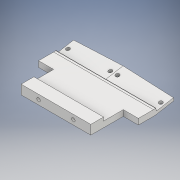
# Autodesk Inventor part: 앞뒷면PSD받침대_수정
Saved by Autodesk Inventor 2017 (Build 210142000, 142)
## iProperties
Part Number: 앞뒷면PSD받침대_수정
Material: ABS 플라스틱
Document SubType Name: Modeling
Designer: minom
Mass: 12.9687 g
Surface Area: 93.8696 cm^2
Volume: 12.2346 cm^3
Density: 1.06 g/cm^3
Appearance: 매끄러움 - 흰색
Author: minom
Autodesk Inventor part; units mm, degrees
ref_plane "YZ Plane" through (0, 0, 0) normal (1, 0, 0) x (0, 1, 0)
ref_plane "XZ Plane" through (0, 0, 0) normal (0, 1, 0) x (-1, 0, 0)
ref_plane "XY Plane" through (0, 0, 0) normal (0, 0, 1) x (1, 0, 0)
sketch "스케치1" plane through (0, 0, 0) normal (0, 0, 1) x (1, 0, 0)
  line L0 (0, 0) -> (60, 0)
  line L1 (60, 0) -> (60, 25)
  line L2 (60, 55) -> (0, 55)
  line L3 (0, 25) -> (0, 0)
  line L4 (-13, 55) -> (73, 55)
  line L5 (73, 55) -> (73, 25)
  line L6 (-13, 25) -> (-13, 55)
  line L7 (73, 25) -> (60, 25)
  line L8 (0, 25) -> (-13, 25)
  dimension "d0" = 60
  dimension "d1" = 55
  dimension "d3" = 86
  dimension "d4" = 30
  dimension "d5" = 13
  constraints: 18 end point, 5 parallel, 2 horizontal, 2 perpendicular
  measures "d0" distance of L2.end L2.start
  measures "d1" distance of L2.start L0.end
  measures "d3" distance of L5.end L6.start
  measures "d4" distance of L4.end L5.end
  measures "d5" distance between parallel lines of L3 L6
extrude "돌출1" add sketch "스케치1" along normal blind 8
sketch "스케치2" plane through (0, 0, 8) normal (0, 0, 1) x (1, 0, 0)
  line L0 (0, 0) -> (60, 0) projected
  line L1 (60, 0) -> (60, 25) projected
  line L2 (60, 25) -> (73, 25) projected
  line L3 (73, 25) -> (73, 55) projected
  line L4 (73, 55) -> (-13, 55) projected
  line L5 (-13, 55) -> (-13, 25) projected
  line L6 (-13, 25) -> (0, 25) projected
  line L7 (0, 25) -> (0, 0) projected
  line L8 (0, 25) -> (0, 0) projected
  line L9 (0, 8) -> (60, 8)
  line L10 (60, 8) -> (60, 0)
  line L11 (60, 0) -> (0, 0)
  line L12 (0, 0) -> (0, 8)
  dimension "d9" = 8
  dimension "d10" = 0
  constraints: 8 end point, 2 parallel, 2 point on line, 1 horizontal, 1 perpendicular
  measures "d9" distance of L9.end L10.end
  measures "d10" distance between parallel lines of L0 L11
extrude "돌출2" cut sketch "스케치2" against normal blind 3 contours L7 L6 L5 L4 L3 L2 L1 L9
sketch "스케치4" plane through (0, 0, 0) normal (0, -1, 0) x (1, 0, 0)
  line L0 (0, 0) -> (60, 0) projected
  line L1 (60, 0) -> (60, 8) projected
  line L2 (0, 8) -> (60, 8) projected
  line L3 (0, 0) -> (0, 8) projected
  circle A0 centre (45, 4) radius 1.5
  circle A1 centre (15, 4) radius 1.5
  dimension "d15" = 3
  dimension "d16" = 3
  dimension "d17" = 4
  dimension "d18" = 15
  dimension "d19" = 4
  dimension "d20" = 15
  constraints: 2 centre point
  measures "d15" diameter of A0
  measures "d16" diameter of A1
  measures "d17" distance from line of L0 A0.centre
  measures "d18" distance from line of L1 A0.centre
  measures "d19" distance from line of L2 A1.centre
  measures "d20" distance from line of L3 A1.centre
extrude "돌출4" cut sketch "스케치4" against normal blind 6 contours A0 | A1
sketch "스케치10" plane through (0, 0, 5) normal (0, 0, 1) x (1, 0, 0)
  line L0 (-10, 38) -> (70, 38)
  line L1 (60, 8) -> (0, 8) projected
  point P0 (0, 0)
  dimension "d42" = 30
  constraints: 2 end point, 1 horizontal
  measures "d42" distance between parallel lines of L1 L0
bend part "굽힘1" radius 10 angle 10 line through (-10, 38, 5) along (1, 0, 0) centre toward (0, 0, 1) moving side (0, 1, 0) both sides no
sketch "스케치11" plane through (-13, 54.7594, 7.8009) normal (0, 0.9848078, 0.1736482) x (1, 0, 0)
  line L0 (0, 0) -> (86, 0) projected
  line L1 (86, 5) -> (86, 0) projected
  line L2 (86, 5) -> (0, 5) projected
  line L3 (0, 5) -> (0, 0) projected
  line L4 (0, 2.5) -> (43, 0)
  line L5 (0, 0) -> (86, 0) projected
  line L6 (73, 2.5147) -> (86, 2.5147) projected
  line L7 (86, 2.5147) -> (43, 0)
  line L8 (43, 0) -> (43, 2.5)
  line L9 (86, 5) -> (0, 5) projected
  line L10 (86, 5) -> (43, 2.5)
  line L11 (0, 5) -> (43, 2.5)
  point P0 (13, -1.8265)
  constraints: 10 end point, 2 midpoint, 1 parallel, 1 perpendicular
extrude "돌출7" cut sketch "스케치11" against normal blind 15 contours L3 L4 L0 | L7 L1 L0 | L11 L2 L10
sketch "스케치12" plane through (30, 54.7594, 7.8009) normal (0.0583814, -0.173352, 0.983128) x (0.9982944, 0.0101378, -0.0574945)
  line L0 (0, 0) -> (43.0735, 0) projected
  line L1 (0, -15) -> (0, 0) projected
  line L2 (0, -15) -> (43.0735, -15) projected
  line L3 (43.0735, 0) -> (43.0735, -15) projected
  circle A0 centre (3.0735, -8) radius 1.6
  circle A1 centre (40.0735, -8) radius 1.6
  point P0 (-30.0555, -55.2821)
  dimension "d47" = 3.2
  dimension "d48" = 3.2
  dimension "d49" = 8
  dimension "d50" = 7
  dimension "d51" = 37
  dimension "d52" = 3
  constraints: 2 centre point
  measures "d47" diameter of A0
  measures "d48" diameter of A1
  measures "d49" distance from line of L0 A0.centre
  measures "d50" distance from line of L2 A1.centre
  measures "d51" distance of A1.centre A0.centre
  measures "d52" distance from line of L3 A1.centre
sketch "스케치13" plane through (-13, 55.1935, 5.3388) normal (-0.0580415, -0.1733554, 0.9831475) x (0.9983142, -0.0100788, 0.0571597)
  circle A0 centre (3, -8) radius 1.6
  circle A1 centre (40, -8) radius 1.6
  line L0 (0, -15) -> (0, 0) projected
  line L1 (0, 0) -> (43.0726, 0) projected
  line L2 (42.9275, -15) -> (-0.1451, -15) projected
  point P0 (13.2292, -55.2821)
  dimension "d53" = 3.2
  dimension "d54" = 3.2
  dimension "d55" = 37
  dimension "d56" = 3
  dimension "d57" = 8
  dimension "d58" = 7
  constraints: 2 centre point
  measures "d53" diameter of A0
  measures "d54" diameter of A1
  measures "d55" distance of A1.centre A0.centre
  measures "d56" distance from line of A0.centre L0
  measures "d57" distance from line of L1 A0.centre
  measures "d58" distance from line of L2 A1.centre
extrude "돌출8" cut sketch "스케치13" against normal blind 3
extrude "돌출9" cut sketch "스케치12" against normal blind 3 contours A0 | A1
sketch "스케치15" plane through (0, 0, 0) normal (0, -1, 0) x (1, 0, 0)
  circle A0 centre (45, 4) radius 1.5 projected
  circle A1 centre (15, 4) radius 1.5 projected
  line L0 (0, 0) -> (60, 0) projected
  line L1 (60, 0) -> (60, 8) projected
  line L2 (0, 8) -> (60, 8) projected
  line L3 (0, 0) -> (0, 8) projected
extrude "돌출11" add sketch "스케치15" along normal blind 3
